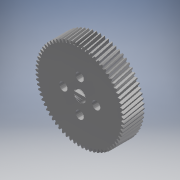
# Autodesk Inventor part: Цилиндрическое зубчатое зацепление1
Saved by Autodesk Inventor 2019 (Build 230136000, 136)
## iProperties
Created: 2019-12-26
Part Number: Цилиндрическое зубчатое зацепление1
Material: Steel
Document SubType Name: Modeling
Designer: Петров Иван
Categories: <?xml version="1.0" encoding="UTF-16"?> <MemberInstance><Categories><FamilyTemplate><FamilyTemplateParameter ValueType="xs:double" Id="1" ObjectReferenceKey="da_z" ObjectType="kUserParameterObject"/><FamilyTemplateParameter ValueType="xs:double" Id="2" ObjectReferenceKey="da_b" ObjectType="kUserParameterObject"/><FamilyTemplateParameter ValueType="xs:double" Id="3" ObjectReferenceKey="da_beta" ObjectType="kUserParameterObject"/><FamilyTemplateParameter ValueType="xs:double" Id="4" ObjectReferenceKey="da_da" ObjectType="kUserParameterObject"/><FamilyTemplateParameter ValueType="xs:double" Id="5" ObjectReferenceKey="da_aw" ObjectType="kUserParameterObject"/><FamilyTemplateParameter ValueType="xs:string" Id="6" ObjectReferenceKey="EAIAABAAAACIAQAAAAAAAIAAAAAAAAAA" ObjectType="83910656" SubObjectId="SurfaceGeometry"/></FamilyTemplate><ParamToTemplateMap><ParamToTemplate CategoryParameter="//CategoryParameter[@InternalName='046C89C9-8512-4d59-83FE-43B91F4F132A']" TemplateParameter="1"/><ParamToTemplate CategoryParameter="//CategoryParameter[@InternalName='2552DF32-E462-4b46-AEBF-C6C7768E72AC']" TemplateParameter="2"/><ParamToTemplate CategoryParameter="//CategoryParameter[@InternalName='C9EE641D-15FC-4fae-A226-E94C4372FDD7']" TemplateParameter="3"/><ParamToTemplate><ParamToTemplate CategoryParameter="//CategoryParameter[@InternalName='00B6519A-459B-49c7-AD84-2E56D39A5744']" ConstantValue="0.000000"/></ParamToTemplate><ParamToTemplate><ParamToTemplate CategoryParameter="//CategoryParameter[@InternalName='04B31F0E-C7A6-4894-AA32-9629BEFACF47']" ConstantValue="1.000000"/></ParamToTemplate><ParamToTemplate><ParamToTemplate CategoryParameter="//CategoryParameter[@InternalName='43CBEC2E-7847-49e7-A936-2F7889FCB2D9']" ConstantValue="0.250000"/></ParamToTemplate><ParamToTemplate><ParamToTemplate CategoryParameter="//CategoryParameter[@InternalName='B1EFC894-105D-4ebd-86BF-FA20ED196853']" ConstantValue="0.350000"/></ParamToTemplate><ParamToTemplate><ParamToTemplate CategoryParameter="//CategoryParameter[@InternalName='51175063-3D10-4879-93E8-6246FE8B403D']" ConstantValue="2060000000.000000"/></ParamToTemplate><ParamToTemplate><ParamToTemplate CategoryParameter="//CategoryParameter[@InternalName='A3A52E27-4454-46a9-B0BD-C932399B70AF']" ConstantValue="0.300000"/></ParamToTemplate><ParamToTemplate><ParamToTemplate CategoryParameter="//CategoryParameter[@InternalName='91B76062-C214-41d9-B1B9-14D2AB99603D']" ConstantValue="0.060000"/></ParamToTemplate><ParamToTemplate><ParamToTemplate CategoryParameter="//CategoryParameter[@InternalName='374E806E-8B8A-4dda-A9AA-1039D6500AD2']" ConstantValue="16.666667"/></ParamToTemplate><ParamToTemplate><ParamToTemplate CategoryParameter="//CategoryParameter[@InternalName='2D373A89-B862-43d6-8D0B-0CBF12AB9F6C']" ConstantValue="0.349066"/></ParamToTemplate><ParamToTemplate CategoryParameter="//CategoryParameter[@InternalName='37777632-D6A2-4fac-9D53-DB8ACD95C989']" TemplateParameter="4"/><ParamToTemplate CategoryParameter="//CategoryParameter[@InternalName='FD1017F1-B727-4f7e-9707-0F86F1FF9423']" TemplateParameter="5"/><ParamToTemplate><ParamToTemplate CategoryParameter="//CategoryParameter[@InternalName='9E1B4470-B2D3-4ff1-B813-535BB4CDF51A']" ConstantValue="3520000.000000"/></ParamToTemplate><ParamToTemplate><ParamToTemplate CategoryParameter="//CategoryParameter[@InternalName='F8452263-BFF6-458c-9FB1-07C4B99E95CD']" ConstantValue="11400000.000000"/></ParamToTemplate><ParamToTemplate><ParamToTemplate CategoryParameter="//CategoryParameter[@InternalName='3E3BB259-FD49-497f-8171-6EBC954A3479']" ConstantValue="2.000000"/></ParamToTemplate><ParamToTemplate CategoryParameter="//CategoryParameter[@InternalName='27C3BAF2-7550-4e4b-AE2C-0DB134B7D9B7']" TemplateParameter="6"/></ParamToTemplateMap><Category DisplayName="Gear" InternalName="DC85795E-93AB-48d5-8EEE-5A27447B64BD" Mnemonic="Gear"><CategoryParameter DisplayName="z" InternalName="046C89C9-8512-4d59-83FE-43B91F4F132A" Mnemonic="z"/><CategoryParameter DisplayName="b" InternalName="2552DF32-E462-4b46-AEBF-C6C7768E72AC" Mnemonic="b"/><CategoryParameter DisplayName="||b|" InternalName="C9EE641D-15FC-4fae-A226-E94C4372FDD7" Mnemonic="beta"/><CategoryParameter DisplayName="x" InternalName="00B6519A-459B-49c7-AD84-2E56D39A5744" Mnemonic="x"/><CategoryParameter DisplayName="a*" InternalName="04B31F0E-C7A6-4894-AA32-9629BEFACF47" Mnemonic="a"/><CategoryParameter DisplayName="c*" InternalName="43CBEC2E-7847-49e7-A936-2F7889FCB2D9" Mnemonic="c"/><CategoryParameter DisplayName="r|.f|*" InternalName="B1EFC894-105D-4ebd-86BF-FA20ED196853" Mnemonic="rf"/><CategoryParameter DisplayName="E" InternalName="51175063-3D10-4879-93E8-6246FE8B403D" Mnemonic="E"/><CategoryParameter DisplayName="||m|" InternalName="A3A52E27-4454-46a9-B0BD-C932399B70AF" Mnemonic="mi"/><Category DisplayName="SpurGear" InternalName="26C5A22E-A91E-4dfd-A3B3-23CCAFAE1764" Mnemonic="SpurGear"><CategoryParameter DisplayName="m" InternalName="91B76062-C214-41d9-B1B9-14D2AB99603D" Mnemonic="m"/><CategoryParameter DisplayName="P" InternalName="374E806E-8B8A-4dda-A9AA-1039D6500AD2" Mnemonic="PP"/><CategoryParameter DisplayName="||a|" InternalName="2D373A89-B862-43d6-8D0B-0CBF12AB9F6C" Mnemonic="alpha"/><CategoryParameter DisplayName="d|.a|" InternalName="37777632-D6A2-4fac-9D53-DB8ACD95C989" Mnemonic="da"/><CategoryParameter DisplayName="a|.w|" InternalName="FD1017F1-B727-4f7e-9707-0F86F1FF9423" Mnemonic="aw"/><CategoryParameter DisplayName="||s||.Flim|" InternalName="9E1B4470-B2D3-4ff1-B813-535BB4CDF51A" Mnemonic="sFlim"/><CategoryParameter DisplayName="||s||.Hlim|" InternalName="F8452263-BFF6-458c-9FB1-07C4B99E95CD" Mnemonic="sHlim"/><CategoryParameter DisplayName="тип" InternalName="3E3BB259-FD49-497f-8171-6EBC954A3479" Mnemonic="type"/><CategoryParameter DisplayName="PitchDiameter" InternalName="27C3BAF2-7550-4e4b-AE2C-0DB134B7D9B7" Mnemonic="IDS_PITCHDIAM"/></Category></Category></Categories></MemberInstance>
Density: 1 g/cm^3
Appearance: Steel
CustomPartVersion: 1
Author: Петров Иван
Autodesk Inventor part; units mm, degrees
ref_plane "YZ Plane" through (0, 0, 0) normal (1, 0, 0) x (0, 1, 0)
ref_plane "XZ Plane" through (0, 0, 0) normal (0, 1, 0) x (-1, 0, 0)
ref_plane "XY Plane" through (0, 0, 0) normal (0, 0, 1) x (1, 0, 0)
sketch "Sketch1" plane through (0, 0, 0) normal (0, 0, 1) x (1, 0, 0)
  circle A0 centre (0, 0) radius 21.6184
  dimension "d0" = 43.2368
  constraints: 1 centre point
  measures "d0" diameter of A0
extrude "Extrusion1" add sketch "Sketch1" along normal blind 10
ref_plane "Work Plane2" through (0, 0, 5) normal (0, 0, 1) x (1, 0, 0)
sketch "Sketch2" plane through (0, 0, 0) normal (0, 0, -1) x (-1, 0, 0)
  circle A0 centre (0, 0) radius 21.6184 projected
  circle A1 centre (0, 0) radius 21.0833
  dimension "d3" = 42.1667
  constraints: 1 centre point, 1 coincident
  measures "d3" diameter of A1
surface extrude "Средний диаметр" sketch "Sketch2" against normal through all shown no curves A1
ref_plane "Work Plane8" through (0, 0, 0) normal (0.9989637, 0.0455146, 0) x (0, 0, 1)
ref_plane "Work Plane9" through (0, 0, 0) normal (1, 0, 0) x (0, 1, 0)
spur gear teeth "Цилиндрическое зубчатое зацепление" teeth 69 pitch diameter 42.0387 tip diameter 43.2368 root diameter 40.5387 face width 10 helix angle 10 hand left start plane through (0, 0, 0) normal (0, 0, -1) x (-1, 0, 0)
sketch "Эскиз3" plane through (0, 0, 10) normal (0, 0, 1) x (1, 0, 0)
  line L0 (0, 0) -> (0, 8)
  circle A0 centre (0, 8) radius 2
  dimension "d49" = 8
  dimension "d50" = 4
  constraints: 2 end point, 1 centre point, 1 coincident, 1 vertical
  measures "d49" distance of L0.start L0.end
  measures "d50" diameter of A0
extrude "Выдавливание2" cut sketch "Эскиз3" against normal through all
sketch "Эскиз4" plane through (0, 0, 0) normal (0, 0, -1) x (-1, 0, 0)
  circle A0 centre (0, 8) radius 2 projected
  circle A1 centre (0, 8) radius 5
  point P0 (0, 0)
  dimension "d61" = 10
  constraints: 1 centre point, 1 coincident
  measures "d61" diameter of A1
extrude "Выдавливание3" cut sketch "Эскиз4" against normal blind 3
pattern_circular "Круговой массив1" count 4 over 360 about axis through (0, 0, 0) along (0, 0, 1) of "Выдавливание2", "Выдавливание3"
sketch "Эскиз5" plane through (0, 0, 0) normal (0, 0, -1) x (-1, 0, 0)
  line L0 (2.8341, 0.75) -> (-2.8341, 0.75)
  line L1 (2.8929, 0.7945) -> (2.8341, 0.75)
  arc A0 (2.8929, 0.7945) -> (2.8468, 0.9465) centre (0, 0) ccw
  line L2 (2.3559, 0.9758) -> (2.8468, 0.9465)
  line L3 (2.6823, 1.3437) -> (2.3559, 0.9758)
  arc A1 (2.6823, 1.3437) -> (2.6074, 1.4837) centre (0, 0) ccw
  line L4 (2.1202, 1.4167) -> (2.6074, 1.4837)
  line L5 (2.3686, 1.8411) -> (2.1202, 1.4167)
  arc A2 (2.3686, 1.8411) -> (2.2678, 1.9639) centre (0, 0) ccw
  line L6 (1.8031, 1.8031) -> (2.2678, 1.9639)
  line L7 (1.9639, 2.2678) -> (1.8031, 1.8031)
  arc A3 (1.9639, 2.2678) -> (1.8411, 2.3686) centre (0, 0) ccw
  line L8 (1.4167, 2.1202) -> (1.8411, 2.3686)
  line L9 (1.4837, 2.6074) -> (1.4167, 2.1202)
  arc A4 (1.4837, 2.6074) -> (1.3437, 2.6823) centre (0, 0) ccw
  line L10 (0.9758, 2.3559) -> (1.3437, 2.6823)
  line L11 (0.9465, 2.8468) -> (0.9758, 2.3559)
  arc A5 (0.9465, 2.8468) -> (0.7945, 2.8929) centre (0, 0) ccw
  line L12 (0.4975, 2.501) -> (0.7945, 2.8929)
  line L13 (0.373, 2.9767) -> (0.4975, 2.501)
  arc A6 (0.373, 2.9767) -> (0.2149, 2.9923) centre (0, 0) ccw
  line L14 (0, 2.55) -> (0.2149, 2.9923)
  line L15 (-0.2149, 2.9923) -> (0, 2.55)
  arc A7 (-0.2149, 2.9923) -> (-0.373, 2.9767) centre (0, 0) ccw
  line L16 (-0.4975, 2.501) -> (-0.373, 2.9767)
  line L17 (-0.7945, 2.8929) -> (-0.4975, 2.501)
  arc A8 (-0.7945, 2.8929) -> (-0.9465, 2.8468) centre (0, 0) ccw
  line L18 (-0.9758, 2.3559) -> (-0.9465, 2.8468)
  line L19 (-1.3437, 2.6823) -> (-0.9758, 2.3559)
  arc A9 (-1.3437, 2.6823) -> (-1.4837, 2.6074) centre (0, 0) ccw
  line L20 (-1.4167, 2.1202) -> (-1.4837, 2.6074)
  line L21 (-1.8411, 2.3686) -> (-1.4167, 2.1202)
  arc A10 (-1.8411, 2.3686) -> (-1.9639, 2.2678) centre (0, 0) ccw
  line L22 (-1.8031, 1.8031) -> (-1.9639, 2.2678)
  line L23 (-2.2678, 1.9639) -> (-1.8031, 1.8031)
  arc A11 (-2.2678, 1.9639) -> (-2.3686, 1.8411) centre (0, 0) ccw
  line L24 (-2.1202, 1.4167) -> (-2.3686, 1.8411)
  line L25 (-2.6074, 1.4837) -> (-2.1202, 1.4167)
  arc A12 (-2.6074, 1.4837) -> (-2.6823, 1.3437) centre (0, 0) ccw
  line L26 (-2.3559, 0.9758) -> (-2.6823, 1.3437)
  line L27 (-2.8468, 0.9465) -> (-2.3559, 0.9758)
  arc A13 (-2.8468, 0.9465) -> (-2.8929, 0.7945) centre (0, 0) ccw
  line L28 (-2.8341, 0.75) -> (-2.8929, 0.7945)
  line L29 (-2.8341, -0.75) -> (2.8341, -0.75)
  line L30 (-2.8929, -0.7945) -> (-2.8341, -0.75)
  arc A14 (-2.8929, -0.7945) -> (-2.8468, -0.9465) centre (0, 0) ccw
  line L31 (-2.3559, -0.9758) -> (-2.8468, -0.9465)
  line L32 (-2.6823, -1.3437) -> (-2.3559, -0.9758)
  arc A15 (-2.6823, -1.3437) -> (-2.6074, -1.4837) centre (0, 0) ccw
  line L33 (-2.1202, -1.4167) -> (-2.6074, -1.4837)
  line L34 (-2.3686, -1.8411) -> (-2.1202, -1.4167)
  arc A16 (-2.3686, -1.8411) -> (-2.2678, -1.9639) centre (0, 0) ccw
  line L35 (-1.8031, -1.8031) -> (-2.2678, -1.9639)
  line L36 (-1.9639, -2.2678) -> (-1.8031, -1.8031)
  arc A17 (-1.9639, -2.2678) -> (-1.8411, -2.3686) centre (0, 0) ccw
  line L37 (-1.4167, -2.1202) -> (-1.8411, -2.3686)
  line L38 (-1.4837, -2.6074) -> (-1.4167, -2.1202)
  arc A18 (-1.4837, -2.6074) -> (-1.3437, -2.6823) centre (0, 0) ccw
  line L39 (-0.9758, -2.3559) -> (-1.3437, -2.6823)
  line L40 (-0.9465, -2.8468) -> (-0.9758, -2.3559)
  arc A19 (-0.9465, -2.8468) -> (-0.7945, -2.8929) centre (0, 0) ccw
  line L41 (-0.4975, -2.501) -> (-0.7945, -2.8929)
  line L42 (-0.373, -2.9767) -> (-0.4975, -2.501)
  arc A20 (-0.373, -2.9767) -> (-0.2149, -2.9923) centre (0, 0) ccw
  line L43 (0, -2.55) -> (-0.2149, -2.9923)
  line L44 (0.2149, -2.9923) -> (0, -2.55)
  arc A21 (0.2149, -2.9923) -> (0.373, -2.9767) centre (0, 0) ccw
  line L45 (0.4975, -2.501) -> (0.373, -2.9767)
  line L46 (0.7945, -2.8929) -> (0.4975, -2.501)
  arc A22 (0.7945, -2.8929) -> (0.9465, -2.8468) centre (0, 0) ccw
  line L47 (0.9758, -2.3559) -> (0.9465, -2.8468)
  line L48 (1.3437, -2.6823) -> (0.9758, -2.3559)
  arc A23 (1.3437, -2.6823) -> (1.4837, -2.6074) centre (0, 0) ccw
  line L49 (1.4167, -2.1202) -> (1.4837, -2.6074)
  line L50 (1.8411, -2.3686) -> (1.4167, -2.1202)
  arc A24 (1.8411, -2.3686) -> (1.9639, -2.2678) centre (0, 0) ccw
  line L51 (1.8031, -1.8031) -> (1.9639, -2.2678)
  line L52 (2.2678, -1.9639) -> (1.8031, -1.8031)
  arc A25 (2.2678, -1.9639) -> (2.3686, -1.8411) centre (0, 0) ccw
  line L53 (2.1202, -1.4167) -> (2.3686, -1.8411)
  line L54 (2.6074, -1.4837) -> (2.1202, -1.4167)
  arc A26 (2.6074, -1.4837) -> (2.6823, -1.3437) centre (0, 0) ccw
  line L55 (2.3559, -0.9758) -> (2.6823, -1.3437)
  line L56 (2.8468, -0.9465) -> (2.3559, -0.9758)
  arc A27 (2.8468, -0.9465) -> (2.8929, -0.7945) centre (0, 0) ccw
  line L57 (2.8341, -0.75) -> (2.8929, -0.7945)
  arc A28 (2.8929, -0.7945) -> (2.8929, 0.7945) centre (0, 0) ccw
  arc A29 (-2.8929, 0.7945) -> (-2.8929, -0.7945) centre (0, 0) ccw
  constraints: 116 end point, 60 point on circle, 30 centre point
extrude "Выдавливание4" cut sketch "Эскиз5" against normal through all contours L0 L28 A13 L27 L26 A12 L25 L24 A11 L23 L22 A10 L21 L20 A9 L19 L18 A8 L17 L16 A7 L15 L14 A6 L13 L12 A5 L11 L10 A4 L9 L8 A3 L7 L6 A2 L5 L4 A1 L3 L2 A0 L1 | A27 L56 L55 A26 L54 L53 A25 L52 L51 A24 L50 L49 A23 L48 L47 A22 L46 L45 A21 L44 L43 A20 L42 L41 A19 L40 L39 A18 L38 L37 A17 L36 L35 A16 L34 L33 A15 L32 L31 A14 L30 L29 L57
equation "\"d0\" = da_da"
equation "\"d1\" = da_b"
equation "\"d3\" = da_dw"
equation "\"d16\" = da_aw"
equation "\"d43\" = da_aw"
equation "\"d46\" = da_aw"
equation "\"da_da\" = 43.23682"
equation "\"da_b\" = 10"
equation "\"da_dw\" = 42.166667"
equation "\"da_aw\" = 27.5"
body "Solid1"
body "Srf1"
